Autodesk Inventor part; units mm, degrees
(part 2 of 2)
sketch "Sketch22" plane through (0, 6.35, 0) normal (0, 1, 0) x (1, 0, 0)
  line L0 (-74.6367, -49.7732) -> (-74.6367, 305.8268) projected
  line L1 (-68.2867, 305.8268) -> (-74.6367, 305.8268)
  line L2 (-74.6367, 305.8268) -> (-74.6367, 280.4268)
  line L3 (-74.6367, 280.4268) -> (-68.2867, 280.4268)
  line L4 (-68.2867, 280.4268) -> (-68.2867, 305.8268)
  line L5 (-68.2867, 280.4268) -> (-74.6367, 280.4268)
  line L6 (-74.6367, 280.4268) -> (-74.6367, 229.6268)
  line L7 (-74.6367, 229.6268) -> (-68.2867, 229.6268)
  line L8 (-68.2867, 229.6268) -> (-68.2867, 280.4268)
  line L9 (-68.2867, 229.6268) -> (-74.6367, 229.6268)
  line L10 (-74.6367, 229.6268) -> (-74.6367, 204.2268)
  line L11 (-74.6367, 204.2268) -> (-68.2867, 204.2268)
  line L12 (-68.2867, 204.2268) -> (-68.2867, 229.6268)
  line L13 (-68.2867, 204.2268) -> (-74.6367, 204.2268)
  line L14 (-74.6367, 204.2268) -> (-74.6367, 153.4268)
  line L15 (-74.6367, 153.4268) -> (-68.2867, 153.4268)
  line L16 (-68.2867, 153.4268) -> (-68.2867, 204.2268)
  line L17 (-68.2867, 153.4268) -> (-74.6367, 153.4268)
  line L18 (-74.6367, 153.4268) -> (-74.6367, 128.0268)
  line L19 (-74.6367, 128.0268) -> (-68.2867, 128.0268)
  line L20 (-68.2867, 128.0268) -> (-68.2867, 153.4268)
  line L21 (-68.2867, 128.0268) -> (-74.6367, 128.0268)
  line L22 (-74.6367, 128.0268) -> (-74.6367, 119.2638)
  line L23 (-74.6367, 119.2638) -> (-68.2867, 119.2638)
  line L24 (-68.2867, 119.2638) -> (-68.2867, 128.0268)
  point P0 (0, 0)
  constraints: 48 end point, 12 parallel, 6 horizontal, 6 perpendicular, 5 point on line, 1 midpoint
extrude "Extrusion21" cut sketch "Sketch22" against normal blind 6.35 contours L0 L19 L24 L23 | L0 L11 L16 L15 | L0 L3 L8 L7
sketch "Sketch23" plane through (0, 6.35, 0) normal (0, 1, 0) x (1, 0, 0)
  line L0 (-68.2867, 204.2268) -> (-68.2867, 153.4268) projected
  line L1 (-68.2867, 119.2638) -> (-42.8867, 119.2638)
  line L2 (-42.8867, 119.2638) -> (-17.4867, 119.2638)
  line L3 (-17.4867, 119.2638) -> (-17.4867, 125.6138)
  line L4 (-17.4867, 125.6138) -> (-42.8867, 125.6138)
  line L5 (-42.8867, 125.6138) -> (-42.8867, 119.2638)
  line L6 (-17.4867, 119.2638) -> (65.0633, 119.2638)
  line L7 (65.0633, 119.2638) -> (90.4633, 119.2638)
  line L8 (90.4633, 119.2638) -> (90.4633, 125.6138)
  line L9 (90.4633, 125.6138) -> (65.0633, 125.6138)
  line L10 (65.0633, 125.6138) -> (65.0633, 119.2638)
  line L11 (90.4633, 119.2638) -> (166.6633, 119.2638)
  line L12 (166.6633, 119.2638) -> (192.0633, 119.2638)
  line L13 (192.0633, 119.2638) -> (192.0633, 125.6138)
  line L14 (192.0633, 125.6138) -> (166.6633, 125.6138)
  line L15 (166.6633, 125.6138) -> (166.6633, 119.2638)
  line L16 (192.0633, 119.2638) -> (268.2633, 119.2638)
  line L17 (268.2633, 119.2638) -> (293.6633, 119.2638)
  line L18 (293.6633, 119.2638) -> (293.6633, 125.6138)
  line L19 (293.6633, 125.6138) -> (268.2633, 125.6138)
  line L20 (268.2633, 125.6138) -> (268.2633, 119.2638)
  line L21 (293.6633, 119.2638) -> (376.2133, 119.2638)
  line L22 (376.2133, 119.2638) -> (401.6133, 119.2638)
  line L23 (401.6133, 119.2638) -> (401.6133, 125.6138)
  line L24 (401.6133, 125.6138) -> (376.2133, 125.6138)
  line L25 (376.2133, 125.6138) -> (376.2133, 119.2638)
  line L26 (65.0633, 125.6138) -> (52.3633, 125.6138)
  line L27 (52.3633, 125.6138) -> (52.3633, 119.2638)
  line L28 (52.3633, 119.2638) -> (65.0633, 119.2638)
  line L29 (65.0633, 119.2638) -> (65.0633, 125.6138)
  line L30 (90.4633, 125.6138) -> (103.1633, 125.6138)
  line L31 (103.1633, 125.6138) -> (103.1633, 119.2638)
  line L32 (103.1633, 119.2638) -> (90.4633, 119.2638)
  line L33 (90.4633, 119.2638) -> (90.4633, 125.6138)
  line L34 (268.2633, 125.6138) -> (255.5633, 125.6138)
  line L35 (255.5633, 125.6138) -> (255.5633, 119.2638)
  line L36 (255.5633, 119.2638) -> (268.2633, 119.2638)
  line L37 (268.2633, 119.2638) -> (268.2633, 125.6138)
  line L38 (293.6633, 125.6138) -> (306.3633, 125.6138)
  line L39 (306.3633, 125.6138) -> (306.3633, 119.2638)
  line L40 (306.3633, 119.2638) -> (293.6633, 119.2638)
  line L41 (293.6633, 119.2638) -> (293.6633, 125.6138)
  point P0 (0, 0)
  dimension "d192" = 25.4
  dimension "d193" = 25.4
  dimension "d194" = 6.35
  dimension "d195" = 82.55
  dimension "d196" = 25.4
  dimension "d197" = 76.2
  dimension "d198" = 25.4
  dimension "d199" = 76.2
  dimension "d200" = 25.4
  dimension "d201" = 82.55
  dimension "d202" = 25.4
  dimension "d203" = 12.7
  dimension "d204" = 12.7
  dimension "d205" = 12.7
  dimension "d206" = 12.7
  constraints: 82 end point, 18 parallel, 14 perpendicular, 9 horizontal, 4 point on line
  measures "d192" distance of L1.start L1.end
  measures "d193" distance of L4.end L3.end
  measures "d194" distance of L3.end L2.end
  measures "d195" distance of L2.end L6.end
  measures "d196" distance of L9.end L8.end
  measures "d197" distance of L7.end L11.end
  measures "d198" distance of L14.end L13.end
  measures "d199" distance of L12.end L16.end
  measures "d200" distance of L19.end L18.end
  measures "d201" distance of L17.end L21.end
  measures "d202" distance of L24.end L23.end
  measures "d203" distance of L28.end L27.end
  measures "d204" distance of L31.end L32.end
  measures "d205" distance of L36.end L35.end
  measures "d206" distance of L39.end L40.end
extrude "Extrusion22" cut sketch "Sketch23" against normal blind 6.35
sketch "Sketch24" plane through (0, 0, 0) normal (0, -1, 0) x (1, 0, 0)
  circle A0 centre (384.8239, -409.6874) radius 1.9812 projected
  circle A1 centre (54.6239, -328.9662) radius 1.9812 projected
  circle A2 centre (304.1027, -79.4874) radius 1.9812 projected
  circle A3 centre (304.1027, 1.2338) radius 1.9812 projected
  circle A4 centre (-26.0973, -328.9662) radius 1.9812 projected
  circle A5 centre (54.6239, -79.4874) radius 1.9812 projected
  circle A6 centre (384.8239, -79.4874) radius 1.9812 projected
  circle A7 centre (54.6239, 1.2338) radius 1.9812 projected
  circle A8 centre (304.1027, -328.9662) radius 1.9812 projected
  circle A9 centre (54.6239, -409.6874) radius 1.9812 projected
  circle A10 centre (-26.0973, -79.4874) radius 1.9812 projected
  circle A11 centre (304.1027, -409.6874) radius 1.9812 projected
  circle A12 centre (384.8239, -328.9662) radius 1.9812 projected
  circle A13 centre (-26.0973, 1.2338) radius 1.9812 projected
  circle A14 centre (-26.0973, -409.6874) radius 1.9812 projected
  circle A15 centre (384.8239, 1.2338) radius 1.9812 projected
  point P0 (0, 0)
extrude "Extrusion23" add sketch "Sketch24" against normal blind 6.35
sketch "Sketch25" plane through (0, 0, 0) normal (0, -1, 0) x (1, 0, 0)
  circle A0 centre (14.2633, -369.3268) radius 19.05 projected
  circle A1 centre (344.4633, -39.1268) radius 19.05 projected
  line L0 (344.4633, -39.1268) -> (384.9509, -39.1268)
  line L1 (384.9509, -39.1268) -> (384.9509, -79.6144)
  line L2 (384.9509, -79.6144) -> (344.4633, -79.6144)
  line L3 (344.4633, -79.6144) -> (344.4633, -39.1268)
  line L4 (384.9509, -79.6144) -> (303.9757, -79.6144)
  line L5 (303.9757, -79.6144) -> (303.9757, 1.3608)
  line L6 (303.9757, 1.3608) -> (384.9509, 1.3608)
  line L7 (384.9509, 1.3608) -> (384.9509, -79.6144)
  line L8 (14.2633, -369.3268) -> (-26.2243, -369.3268)
  line L9 (-26.2243, -369.3268) -> (-26.2243, -409.8144)
  line L10 (-26.2243, -409.8144) -> (14.2633, -409.8144)
  line L11 (14.2633, -409.8144) -> (14.2633, -369.3268)
  line L12 (-26.2243, -409.8144) -> (54.7509, -409.8144)
  line L13 (54.7509, -409.8144) -> (54.7509, -328.8392)
  line L14 (54.7509, -328.8392) -> (-26.2243, -328.8392)
  line L15 (-26.2243, -328.8392) -> (-26.2243, -409.8144)
  line L16 (384.9509, -328.8392) -> (303.9757, -328.8392)
  line L17 (303.9757, -328.8392) -> (303.9757, -409.8144)
  line L18 (303.9757, -409.8144) -> (384.9509, -409.8144)
  line L19 (384.9509, -409.8144) -> (384.9509, -328.8392)
  line L20 (54.7509, -79.6144) -> (-26.2243, -79.6144)
  line L21 (-26.2243, -79.6144) -> (-26.2243, 1.3608)
  line L22 (-26.2243, 1.3608) -> (54.7509, 1.3608)
  line L23 (54.7509, 1.3608) -> (54.7509, -79.6144)
  circle A2 centre (384.9509, 1.3608) radius 1.9812
  circle A3 centre (384.9509, -79.6144) radius 1.9812
  circle A4 centre (303.9757, -79.6144) radius 1.9812
  circle A5 centre (303.9757, 1.3608) radius 1.9812
  circle A6 centre (54.7509, 1.3608) radius 1.9812
  circle A7 centre (54.7509, -79.6144) radius 1.9812
  circle A8 centre (-26.2243, -79.6144) radius 1.9812
  circle A9 centre (-26.2243, 1.3608) radius 1.9812
  circle A10 centre (54.7509, -328.8392) radius 1.9812
  circle A11 centre (54.7509, -409.8144) radius 1.9812
  circle A12 centre (-26.2243, -409.8144) radius 1.9812
  circle A13 centre (-26.2243, -328.8392) radius 1.9812
  circle A14 centre (384.9509, -328.8392) radius 1.9812
  circle A15 centre (303.9757, -328.8392) radius 1.9812
  circle A16 centre (303.9757, -409.8144) radius 1.9812
  circle A17 centre (384.9509, -409.8144) radius 1.9812
  point P0 (0, 0)
  dimension "d211" = 40.4876
  dimension "d212" = 40.4876
  dimension "d213" = 80.9752
  dimension "d214" = 80.9752
  dimension "d215" = 40.4876
  dimension "d216" = 40.4876
  dimension "d217" = 80.9752
  dimension "d218" = 80.9752
  dimension "d219" = 3.9624
  dimension "d220" = 3.9624
  dimension "d221" = 3.9624
  dimension "d222" = 3.9624
  dimension "d223" = 3.9624
  dimension "d224" = 3.9624
  dimension "d225" = 3.9624
  dimension "d226" = 3.9624
  dimension "d227" = 3.9624
  dimension "d228" = 3.9624
  dimension "d229" = 3.9624
  dimension "d230" = 3.9624
  dimension "d231" = 3.9624
  dimension "d232" = 3.9624
  dimension "d233" = 3.9624
  dimension "d234" = 3.9624
  constraints: 48 end point, 16 centre point, 16 coincident, 12 parallel, 6 horizontal, 6 perpendicular
  measures "d211" distance of L1.end L2.end
  measures "d212" distance of L0.end L1.end
  measures "d213" distance of L5.end L6.end
  measures "d214" distance of L4.end L5.end
  measures "d215" distance of L10.end L9.end
  measures "d216" distance of L9.end L8.end
  measures "d217" distance of L14.end L13.end
  measures "d218" distance of L13.end L12.end
  measures "d219" diameter of A2
  measures "d220" diameter of A3
  measures "d221" diameter of A4
  measures "d222" diameter of A5
  measures "d223" diameter of A6
  measures "d224" diameter of A7
  measures "d225" diameter of A8
  measures "d226" diameter of A9
  measures "d227" diameter of A10
  measures "d228" diameter of A11
  measures "d229" diameter of A12
  measures "d230" diameter of A13
  measures "d231" diameter of A14
  measures "d232" diameter of A15
  measures "d233" diameter of A16
  measures "d234" diameter of A17
extrude "Extrusion24" cut sketch "Sketch25" against normal blind 6.35 contours A12 L10 L9 | L9 L10 A12 | A13 L14 L15 | L15 L14 A13 | A11 L13 L12 | L12 L13 A11 | A10 L13 L14 | L14 L13 A10 | A3 L2 L1 | L1 L2 A3 | A2 L6 L7 | L7 L6 A2 | A4 L5 L4 | L4 L5 A4 | A5 L5 L6 | L6 L5 A5 | A15 L17 L16 | L16 L17 A15 | A14 L19 L16 | L16 L19 A14 | A16 L18 L17 | L17 L18 A16 | A17 L18 L19 | L19 L18 A17 | A8 L21 L20 | L20 L21 A8 | A7 L23 L20 | L20 L23 A7 | A9 L22 L21 | L21 L22 A9 | A6 L22 L23 | L23 L22 A6
sketch "Sketch26" plane through (0, 6.35, 0) normal (0, 1, 0) x (1, 0, 0)
  line L0 (401.6133, 125.6138) -> (401.6133, 119.2638) projected
  line L1 (401.6133, 119.2638) -> (376.2133, 119.2638) projected
  line L2 (376.2133, 119.2638) -> (376.2133, 125.6138) projected
  line L3 (376.2133, 125.6138) -> (401.6133, 125.6138) projected
  line L4 (52.3633, 119.2638) -> (52.3633, 125.6138) projected
  line L5 (52.3633, 125.6138) -> (103.1633, 125.6138) projected
  line L6 (103.1633, 125.6138) -> (103.1633, 119.2638) projected
  line L7 (103.1633, 119.2638) -> (52.3633, 119.2638) projected
  line L8 (255.5633, 119.2638) -> (255.5633, 125.6138) projected
  line L9 (255.5633, 125.6138) -> (306.3633, 125.6138) projected
  line L10 (306.3633, 125.6138) -> (306.3633, 119.2638) projected
  line L11 (306.3633, 119.2638) -> (255.5633, 119.2638) projected
  line L12 (192.0633, 125.6138) -> (192.0633, 119.2638) projected
  line L13 (192.0633, 119.2638) -> (166.6633, 119.2638) projected
  line L14 (166.6633, 119.2638) -> (166.6633, 125.6138) projected
  line L15 (166.6633, 125.6138) -> (192.0633, 125.6138) projected
  line L16 (-17.4867, 125.6138) -> (-17.4867, 119.2638) projected
  line L17 (-17.4867, 119.2638) -> (-42.8867, 119.2638) projected
  line L18 (-42.8867, 119.2638) -> (-42.8867, 125.6138) projected
  line L19 (-42.8867, 125.6138) -> (-17.4867, 125.6138) projected
  line L20 (433.3633, 119.2638) -> (420.6633, 119.2638)
  line L21 (420.6633, 119.2638) -> (420.6633, 458.2268)
  line L22 (420.6633, 458.2268) -> (433.3633, 458.2268)
  line L23 (433.3633, 458.2268) -> (433.3633, 119.2638)
  line L24 (420.6633, 458.2268) -> (-74.6367, 458.2268)
  line L25 (-74.6367, 458.2268) -> (-74.6367, 445.5268)
  line L26 (-74.6367, 445.5268) -> (420.6633, 445.5268)
  line L27 (420.6633, 445.5268) -> (420.6633, 458.2268)
  line L28 (-74.6367, 458.2268) -> (-68.2867, 458.2268)
  line L29 (-68.2867, 458.2268) -> (-68.2867, 119.2638)
  line L30 (-68.2867, 119.2638) -> (-74.6367, 119.2638)
  line L31 (-74.6367, 119.2638) -> (-74.6367, 458.2268)
  line L32 (-68.2867, 119.2638) -> (433.3633, 119.2638)
  line L33 (433.3633, 119.2638) -> (433.3633, 128.0268)
  line L34 (433.3633, 128.0268) -> (-68.2867, 128.0268)
  line L35 (-68.2867, 128.0268) -> (-68.2867, 119.2638)
  point P0 (0, 0)
  constraints: 32 end point, 8 parallel, 4 horizontal, 4 perpendicular
extrude "Extrusion25" add sketch "Sketch26" against normal blind 6.35 contours L0 L1 L2 L3 | L21 L34 L23 L20 | L11 L8 L9 L10 | L21 L22 L23 L34 | L26 L29 L24 L21 | L29 L30 L31 L26 | L13 L14 L15 L12 | L26 L25 L24 L29 | L18 L19 L16 L17 | L7 L4 L5 L6
sketch "Sketch27" plane through (0, 6.35, 0) normal (0, 1, 0) x (1, 0, 0)
  line L0 (258.1033, -43.4232) -> (100.6233, -43.4232)
  line L1 (100.6233, -43.4232) -> (100.6233, -49.7732)
  line L2 (100.6233, -49.7732) -> (258.1033, -49.7732)
  line L3 (258.1033, -49.7732) -> (258.1033, -43.4232)
  point P0 (0, 0)
  constraints: 8 end point, 2 parallel, 1 horizontal, 1 perpendicular
extrude "Extrusion26" add sketch "Sketch27" against normal blind 6.35
sketch "Sketch28" plane through (0, 6.35, 0) normal (0, 1, 0) x (1, 0, 0)
  circle A0 centre (14.2633, 369.3268) radius 19.05 projected
  circle A1 centre (14.2633, 39.1268) radius 19.05 projected
  circle A2 centre (344.4633, 369.3268) radius 19.05 projected
  circle A3 centre (344.4633, 39.1268) radius 19.05 projected
  circle A4 centre (54.7509, 328.8392) radius 1.9812 projected
  circle A5 centre (303.9757, 79.6144) radius 1.9812 projected
  circle A6 centre (384.9509, 79.6144) radius 1.9812 projected
  circle A7 centre (384.9509, 328.8392) radius 1.9812 projected
  circle A8 centre (54.7509, 409.8144) radius 1.9812 projected
  circle A9 centre (-26.2243, 328.8392) radius 1.9812 projected
  circle A10 centre (303.9757, -1.3608) radius 1.9812 projected
  circle A11 centre (54.7509, -1.3608) radius 1.9812 projected
  circle A12 centre (-26.2243, 79.6144) radius 1.9812 projected
  circle A13 centre (384.9509, -1.3608) radius 1.9812 projected
  circle A14 centre (-26.2243, -1.3608) radius 1.9812 projected
  circle A15 centre (54.7509, 79.6144) radius 1.9812 projected
  circle A16 centre (-26.2243, 409.8144) radius 1.9812 projected
  circle A17 centre (303.9757, 328.8392) radius 1.9812 projected
  circle A18 centre (303.9757, 409.8144) radius 1.9812 projected
  circle A19 centre (384.9509, 409.8144) radius 1.9812 projected
  line L0 (433.3633, -49.7732) -> (-74.6367, -49.7732) projected
  line L1 (433.3633, 458.2268) -> (433.3633, -49.7732) projected
  line L2 (-74.6367, 458.2268) -> (433.3633, 458.2268) projected
  line L3 (-74.6367, -49.7732) -> (-74.6367, 458.2268) projected
  point P0 (0, 0)
extrude "Extrusion27" add sketch "Sketch28" along normal blind 6.35
sketch "Sketch29" plane through (0, 12.7, 0) normal (0, 1, 0) x (1, 0, 0)
  line L0 (433.3633, -49.7732) -> (-74.6367, -49.7732) projected
  line L1 (-74.6367, -49.7732) -> (94.2733, -49.7732)
  line L2 (94.2733, -49.7732) -> (264.4533, -49.7732)
  line L3 (94.2733, -49.7732) -> (264.4533, -49.7732)
  line L4 (264.4533, -49.7732) -> (264.4533, -37.0732)
  line L5 (264.4533, -37.0732) -> (94.2733, -37.0732)
  line L6 (94.2733, -37.0732) -> (94.2733, -49.7732)
  point P0 (0, 0)
  dimension "d243" = 168.91
  dimension "d244" = 170.18
  dimension "d245" = 12.7
  constraints: 12 end point, 2 parallel, 2 point on line, 1 horizontal, 1 perpendicular
  measures "d243" distance of L0.end L1.end
  measures "d244" distance of L1.end L2.end
  measures "d245" distance of L4.end L3.end
extrude "Extrusion28" cut sketch "Sketch29" against normal blind 12.7
sketch "Sketch30" plane through (0, 12.7, 0) normal (0, 1, 0) x (1, 0, 0)
  line L0 (94.2733, -37.0732) -> (264.4533, -37.0732) projected
  line L1 (94.2733, -37.0732) -> (106.9733, -37.0732)
  line L2 (264.4533, -37.0732) -> (251.7533, -37.0732)
  line L3 (106.9733, -37.0732) -> (251.7533, -37.0732)
  line L4 (251.7533, -37.0732) -> (251.7533, -49.7732)
  line L5 (251.7533, -49.7732) -> (106.9733, -49.7732)
  line L6 (106.9733, -49.7732) -> (106.9733, -37.0732)
  point P0 (0, 0)
  dimension "d248" = 12.7
  dimension "d249" = 12.7
  dimension "d250" = 12.7
  constraints: 12 end point, 2 parallel, 2 point on line, 1 horizontal, 1 perpendicular
  measures "d248" distance of L0.start L1.end
  measures "d249" distance of L0.end L2.end
  measures "d250" distance of L3.end L4.end
extrude "Extrusion29" add sketch "Sketch30" against normal blind 12.7
sketch "Sketch31" plane through (0, 12.7, 0) normal (0, 1, 0) x (1, 0, 0)
  line L0 (264.4533, -37.0732) -> (264.4533, -49.7732) projected
  line L1 (433.3633, -49.7732) -> (264.4533, -49.7732) projected
  line L2 (94.2733, -49.7732) -> (-74.6367, -49.7732) projected
  line L3 (94.2733, -37.0732) -> (87.9233, -37.0732)
  line L4 (87.9233, -37.0732) -> (87.9233, -49.7732)
  line L5 (87.9233, -49.7732) -> (94.2733, -49.7732)
  line L6 (94.2733, -49.7732) -> (94.2733, -37.0732)
  line L7 (264.4533, -37.0732) -> (270.8033, -37.0732)
  line L8 (270.8033, -37.0732) -> (270.8033, -49.7732)
  line L9 (270.8033, -49.7732) -> (264.4533, -49.7732)
  line L10 (264.4533, -49.7732) -> (264.4533, -37.0732)
  point P0 (0, 0)
  dimension "d253" = 6.35
  dimension "d254" = 6.35
  constraints: 16 end point, 4 parallel, 2 horizontal, 2 perpendicular, 2 point on line
  measures "d253" distance of L5.end L4.end
  measures "d254" distance of L8.end L9.end
extrude "Extrusion30" cut sketch "Sketch31" against normal blind 12.7
sketch "Sketch32" plane through (0, 12.7, 0) normal (0, 1, 0) x (1, 0, 0)
  line L0 (270.8033, -37.0732) -> (270.8033, -49.7732) projected
  line L1 (433.3633, -49.7732) -> (270.8033, -49.7732) projected
  line L2 (270.8033, -37.0732) -> (277.1533, -37.0732)
  line L3 (277.1533, -37.0732) -> (277.1533, -49.7732)
  line L4 (277.1533, -49.7732) -> (270.8033, -49.7732)
  line L5 (270.8033, -49.7732) -> (270.8033, -37.0732)
  point P0 (0, 0)
  dimension "d257" = 6.35
  constraints: 8 end point, 2 parallel, 1 horizontal, 1 perpendicular, 1 point on line
  measures "d257" distance of L3.end L4.end
extrude "Extrusion31" cut sketch "Sketch32" against normal blind 12.7
sketch "Sketch33" plane through (0, 12.7, 0) normal (0, 1, 0) x (1, 0, 0)
  line L0 (251.7533, -37.0732) -> (277.1533, -37.0732) projected
  line L1 (277.1533, -49.7732) -> (270.8033, -49.7732)
  line L2 (270.8033, -49.7732) -> (270.8033, -37.0732)
  line L3 (270.8033, -37.0732) -> (277.1533, -37.0732)
  line L4 (277.1533, -37.0732) -> (277.1533, -49.7732)
  point P0 (0, 0)
  dimension "d260" = 6.35
  constraints: 8 end point, 2 parallel, 1 horizontal, 1 perpendicular, 1 point on line
  measures "d260" distance of L2.end L3.end
extrude "Extrusion32" add sketch "Sketch33" against normal blind 12.7
sketch "Sketch34" plane through (0, 12.7, 0) normal (0, 1, 0) x (1, 0, 0)
  line L0 (433.3633, -49.7732) -> (270.8033, -49.7732) projected
  line L1 (87.9233, -49.7732) -> (-74.6367, -49.7732) projected
  line L2 (87.9233, -37.0732) -> (81.5733, -37.0732)
  line L3 (81.5733, -37.0732) -> (81.5733, -49.7732)
  line L4 (81.5733, -49.7732) -> (87.9233, -49.7732)
  line L5 (87.9233, -49.7732) -> (87.9233, -37.0732)
  line L6 (270.8033, -37.0732) -> (277.1533, -37.0732)
  line L7 (277.1533, -37.0732) -> (277.1533, -49.7732)
  line L8 (277.1533, -49.7732) -> (270.8033, -49.7732)
  line L9 (270.8033, -49.7732) -> (270.8033, -37.0732)
  point P0 (0, 0)
  dimension "d263" = 6.35
  dimension "d264" = 6.35
  constraints: 16 end point, 4 parallel, 2 horizontal, 2 perpendicular, 2 point on line
  measures "d263" distance of L4.end L3.end
  measures "d264" distance of L7.end L8.end
extrude "Extrusion33" cut sketch "Sketch34" against normal blind 12.7
sketch "Sketch35" plane through (0, 12.7, 0) normal (0, 1, 0) x (1, 0, 0)
  line L0 (433.3633, 458.2268) -> (433.3633, -49.7732) projected
  line L1 (-74.6367, 458.2268) -> (433.3633, 458.2268) projected
  line L2 (-74.6367, -49.7732) -> (-74.6367, 458.2268) projected
  line L3 (433.3633, 204.2268) -> (433.3633, 302.0168)
  line L4 (433.3633, 302.0168) -> (433.3633, 106.4368)
  line L5 (433.3633, 106.4368) -> (420.6633, 106.4368)
  line L6 (420.6633, 106.4368) -> (420.6633, 131.8368)
  line L7 (420.6633, 131.8368) -> (433.3633, 131.8368)
  line L8 (433.3633, 131.8368) -> (433.3633, 106.4368)
  line L9 (433.3633, 302.0168) -> (420.6633, 302.0168)
  line L10 (420.6633, 302.0168) -> (420.6633, 276.6168)
  line L11 (420.6633, 276.6168) -> (433.3633, 276.6168)
  line L12 (433.3633, 276.6168) -> (433.3633, 302.0168)
  line L13 (251.7533, 458.2268) -> (277.1533, 458.2268)
  line L14 (277.1533, 458.2268) -> (277.1533, 445.5268)
  line L15 (277.1533, 445.5268) -> (251.7533, 445.5268)
  line L16 (251.7533, 445.5268) -> (251.7533, 458.2268)
  line L17 (106.9733, 445.5268) -> (81.5733, 445.5268)
  line L18 (81.5733, 445.5268) -> (81.5733, 458.2268)
  line L19 (81.5733, 458.2268) -> (106.9733, 458.2268)
  line L20 (106.9733, 458.2268) -> (106.9733, 445.5268)
  line L21 (-74.6367, 302.0168) -> (-61.9367, 302.0168)
  line L22 (-61.9367, 302.0168) -> (-61.9367, 276.6168)
  line L23 (-61.9367, 276.6168) -> (-74.6367, 276.6168)
  line L24 (-74.6367, 276.6168) -> (-74.6367, 302.0168)
  line L25 (-74.6367, 106.4368) -> (-61.9367, 106.4368)
  line L26 (-61.9367, 106.4368) -> (-61.9367, 131.8368)
  line L27 (-61.9367, 131.8368) -> (-74.6367, 131.8368)
  line L28 (-74.6367, 131.8368) -> (-74.6367, 106.4368)
  point P0 (0, 0)
  dimension "d267" = 97.79
  dimension "d268" = 195.58
  dimension "d269" = 12.7
  dimension "d270" = 25.4
  dimension "d271" = 25.4
  dimension "d272" = 12.7
  dimension "d273" = 12.7
  constraints: 52 end point, 12 parallel, 6 horizontal, 6 perpendicular, 6 point on line, 1 midpoint
  measures "d267" distance of L3.start L3.end
  measures "d268" distance of L3.end L4.end
  measures "d269" distance of L6.end L7.end
  measures "d270" distance of L5.end L6.end
  measures "d271" distance of L10.end L9.end
  measures "d272" distance of L13.end L14.end
  measures "d273" distance of L22.end L23.end
extrude "Extrusion34" cut sketch "Sketch35" against normal blind 25.4
sketch "Sketch36" plane through (0, 0, 0) normal (0, -1, 0) x (1, 0, 0)
  line L0 (-74.6367, 49.7732) -> (153.9633, 49.7732)
  line L1 (153.9633, 49.7732) -> (153.9633, -145.8068)
  line L2 (153.9633, -145.8068) -> (-74.6367, -145.8068)
  line L3 (-74.6367, -145.8068) -> (-74.6367, 49.7732)
  line L4 (153.9633, -145.8068) -> (141.2633, -145.8068)
  line L5 (141.2633, -145.8068) -> (141.2633, -120.4068)
  line L6 (141.2633, -120.4068) -> (153.9633, -120.4068)
  line L7 (153.9633, -120.4068) -> (153.9633, -145.8068)
  line L8 (433.3633, 49.7732) -> (204.7633, 49.7732)
  line L9 (204.7633, 49.7732) -> (204.7633, -145.8068)
  line L10 (204.7633, -145.8068) -> (433.3633, -145.8068)
  line L11 (433.3633, -145.8068) -> (433.3633, 49.7732)
  line L12 (204.7633, -145.8068) -> (217.4633, -145.8068)
  line L13 (217.4633, -145.8068) -> (217.4633, -120.4068)
  line L14 (217.4633, -120.4068) -> (204.7633, -120.4068)
  line L15 (204.7633, -120.4068) -> (204.7633, -145.8068)
  point P0 (0, 0)
  dimension "d276" = 228.6
  dimension "d277" = 195.58
  dimension "d278" = 12.7
  dimension "d279" = 25.4
  dimension "d280" = 228.6
  dimension "d281" = 12.7
  constraints: 32 end point, 8 parallel, 4 horizontal, 4 perpendicular
  measures "d276" distance of L1.end L2.end
  measures "d277" distance of L0.end L1.end
  measures "d278" distance of L5.end L6.end
  measures "d279" distance of L4.end L5.end
  measures "d280" distance of L10.end L9.end
  measures "d281" distance of L14.end L13.end
extrude "Extrusion35" cut sketch "Sketch36" against normal blind 25.4 contours L1 L2 L5 L6 | L14 L13 L10 L9
sketch "Sketch37" plane through (0, 12.7, 0) normal (0, 1, 0) x (1, 0, 0)
  line L0 (-74.6367, 458.2268) -> (-36.5367, 458.2268)
  line L1 (-36.5367, 458.2268) -> (-36.5367, 432.8268)
  line L2 (-36.5367, 432.8268) -> (-74.6367, 432.8268)
  line L3 (-74.6367, 432.8268) -> (-74.6367, 458.2268)
  circle A0 centre (-36.5367, 432.8268) radius 1.9812
  line L4 (433.3633, 458.2268) -> (395.2633, 458.2268)
  line L5 (395.2633, 458.2268) -> (395.2633, 432.8268)
  line L6 (395.2633, 432.8268) -> (433.3633, 432.8268)
  line L7 (433.3633, 432.8268) -> (433.3633, 458.2268)
  circle A1 centre (395.2633, 432.8268) radius 1.9812
  point P0 (0, 0)
  dimension "d54" = 38.1
  dimension "d284" = 38.1
  dimension "d285" = 25.4
  dimension "d286" = 3.9624
  dimension "d287" = 38.1
  dimension "d288" = 25.4
  dimension "d289" = 3.9624
  constraints: 16 end point, 4 parallel, 2 centre point, 2 coincident, 2 horizontal, 2 perpendicular
  measures "d284" distance of L1.end L2.end
  measures "d285" distance of L0.end L1.end
  measures "d286" diameter of A0
  measures "d287" distance of L6.end L5.end
  measures "d288" distance of L5.end L4.end
  measures "d289" diameter of A1
extrude "Extrusion36" cut sketch "Sketch37" against normal blind 25.4 contours A0 L2 L1 | L1 L2 A0 | A1 L6 L5 | L5 L6 A1
sketch "Sketch38" plane through (0, 12.7, 0) normal (0, 1, 0) x (1, 0, 0)
  circle A0 centre (-36.5367, 432.8268) radius 1.9812 projected
  circle A1 centre (395.2633, 432.8268) radius 1.9812 projected
  line L0 (277.1533, 445.5268) -> (251.7533, 445.5268) projected
  line L1 (-36.5367, 432.8268) -> (-36.5367, 169.9368)
  line L2 (395.2633, 432.8268) -> (395.2633, 169.9368)
  line L3 (395.2633, 169.9368) -> (369.8633, 169.9368)
  line L4 (369.8633, 169.9368) -> (369.8633, 195.3368)
  line L5 (369.8633, 195.3368) -> (395.2633, 195.3368)
  line L6 (395.2633, 195.3368) -> (395.2633, 169.9368)
  line L7 (-36.5367, 169.9368) -> (-11.1367, 169.9368)
  line L8 (-11.1367, 169.9368) -> (-11.1367, 195.3368)
  line L9 (-11.1367, 195.3368) -> (-36.5367, 195.3368)
  line L10 (-36.5367, 195.3368) -> (-36.5367, 169.9368)
  circle A2 centre (369.8633, 195.3368) radius 1.9812
  circle A3 centre (-11.1367, 195.3368) radius 1.9812
  point P0 (0, 0)
  dimension "d292" = 262.89
  dimension "d293" = 25.4
  dimension "d294" = 25.4
  dimension "d295" = 25.4
  dimension "d296" = 25.4
  dimension "d297" = 3.9624
  dimension "d298" = 3.9624
  constraints: 20 end point, 5 parallel, 3 perpendicular, 2 centre point, 2 coincident, 2 horizontal
  measures "d292" distance of L1.start L1.end
  measures "d293" distance of L4.end L5.end
  measures "d294" distance of L3.end L4.end
  measures "d295" distance of L9.end L8.end
  measures "d296" distance of L8.end L7.end
  measures "d297" diameter of A2
  measures "d298" diameter of A3
extrude "Extrusion37" cut sketch "Sketch38" against normal blind 25.4 contours A3 L8 L9 | L9 L8 A3 | A2 L4 L5 | L5 L4 A2
sketch "Sketch39" plane through (0, 0, 0) normal (0, -1, 0) x (1, 0, 0)
  line L0 (251.7533, -458.2268) -> (106.9733, -458.2268) projected
  line L1 (179.3633, -458.2268) -> (179.3633, -450.2268)
  circle A0 centre (179.3633, -450.2268) radius 5
  line L2 (179.3633, -458.2268) -> (179.3633, -428.2268)
  circle A1 centre (179.3633, -428.2268) radius 5
  point P0 (0, 0)
  dimension "d301" = 8
  dimension "d302" = 10
  dimension "d303" = 30
  constraints: 4 end point, 2 centre point, 2 coincident, 1 collinear, 1 midpoint, 1 perpendicular
  measures "d301" distance of L1.start L1.end
  measures "d302" diameter of A0
  measures "d303" distance of L1.start L2.end
extrude "Extrusion38" cut sketch "Sketch39" against normal blind 25.4
sketch "Sketch40" plane through (0, 12.7, 0) normal (0, 1, 0) x (1, 0, 0)
  line L0 (106.9733, -49.7732) -> (251.7533, -49.7732) projected
  line L1 (277.1533, 445.5268) -> (251.7533, 445.5268) projected
  line L2 (179.3633, -49.7732) -> (179.3633, 60.2268)
  line L3 (179.3633, 60.2268) -> (157.8633, 60.2268)
  line L4 (157.8633, 60.2268) -> (200.8633, 60.2268)
  line L5 (179.3633, 60.2268) -> (179.3633, 65.2268)
  circle A0 centre (179.3633, 65.2268) radius 15.875
  line L6 (179.3633, 65.2268) -> (179.3633, 67.7268)
  circle A1 centre (179.3633, 67.7268) radius 15.875
  line L7 (163.4883, 67.7268) -> (163.4883, 65.2268)
  line L8 (195.2383, 65.2268) -> (195.2383, 67.7268)
  circle A2 centre (157.8633, 60.2268) radius 1.9812
  circle A3 centre (200.8633, 60.2268) radius 1.9812
  point P0 (0, 0)
  dimension "d306" = 110
  dimension "d307" = 21.5
  dimension "d308" = 43
  dimension "d309" = 5
  dimension "d310" = 31.75
  dimension "d311" = 2.5
  dimension "d312" = 3.9624
  dimension "d313" = 3.9624
  constraints: 14 end point, 4 centre point, 4 coincident, 4 point on circle, 3 perpendicular, 3 tangent, 1 collinear, 1 midpoint, 1 point on line
  measures "d306" distance of L2.start L2.end
  measures "d307" distance of L2.end L3.end
  measures "d308" distance of L3.end L4.end
  measures "d309" distance of L2.end L5.end
  measures "d310" diameter of A0
  measures "d311" distance of L6.start L6.end
  measures "d312" diameter of A2
  measures "d313" diameter of A3
extrude "Extrusion39" cut sketch "Sketch40" against normal blind 25.4
body "Solid1"
